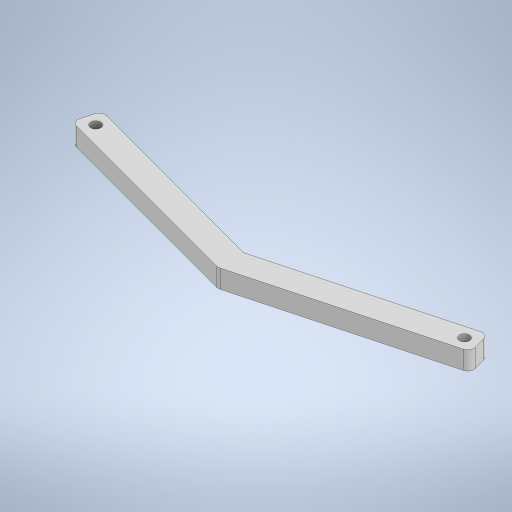
# Autodesk Inventor part: Part3
Saved by Autodesk Inventor 2023 (Build 270158000, 158)
## iProperties
Created: 2023-03-01
Part Number: Part3
Material: Generic
Document SubType Name: Modeling
Designer: Gabriel - T3 CAD
Density: 1 g/cm^3
Appearance: Default
Author: Gabriel - T3 CAD
Autodesk Inventor part; units mm, degrees
ref_plane "YZ Plane" through (0, 0, 0) normal (1, 0, 0) x (0, 1, 0)
ref_plane "XZ Plane" through (0, 0, 0) normal (0, 1, 0) x (-1, 0, 0)
ref_plane "XY Plane" through (0, 0, 0) normal (0, 0, 1) x (1, 0, 0)
sketch "Sketch1" plane through (0, 0, 0) normal (0, 1, 0) x (-1, 0, 0)
  line L0 (0, 0) -> (190.5, 0)
  line L1 (190.5, 0) -> (95.25, 25.5222)
  line L2 (95.25, 25.5222) -> (0, 0)
  line L3 (95.25, 0) -> (95.25, 153.3461)
  line L4 (1.6435, -6.1336) -> (-1.6435, 6.1336)
  line L5 (-1.6435, 6.1336) -> (94.4282, 31.876)
  line L6 (94.4282, 18.728) -> (1.6435, -6.1336)
  line L7 (45.4353, 45.444) -> (42.1483, 33.1767)
  line L8 (96.0718, 18.728) -> (188.8565, -6.1336)
  line L9 (188.8565, -6.1336) -> (192.1435, 6.1336)
  line L10 (192.1435, 6.1336) -> (96.0718, 31.876)
  arc A0 (96.0718, 31.876) -> (94.4282, 31.876) centre (95.25, 28.8092) ccw
  arc A1 (96.0718, 18.728) -> (94.4282, 18.728) centre (95.25, 15.6612) ccw
  circle A2 centre (95.25, 25.5222) radius 2.5797
  circle A3 centre (190.5, 0) radius 2.5797
  circle A4 centre (0, 0) radius 2.5797
  line L11 (192.1435, 6.1336) -> (188.8565, -6.1336)
  line L12 (188.8565, -6.1336) -> (191.9233, -6.9554)
  line L13 (195.8119, -4.7103) -> (197.4554, 1.4233)
  line L14 (195.2103, 5.3119) -> (192.1435, 6.1336)
  arc A5 (197.4554, 1.4233) -> (195.2103, 5.3119) centre (194.3886, 2.2451) ccw
  arc A6 (191.9233, -6.9554) -> (195.8119, -4.7103) centre (192.7451, -3.8886) ccw
  line L15 (-1.6435, 6.1336) -> (1.6435, -6.1336)
  line L16 (1.6435, -6.1336) -> (-1.4233, -6.9554)
  line L17 (-5.3119, -4.7103) -> (-6.9554, 1.4233)
  line L18 (-4.7103, 5.3119) -> (-1.6435, 6.1336)
  arc A7 (-4.7103, 5.3119) -> (-6.9554, 1.4233) centre (-3.8886, 2.2451) ccw
  arc A8 (-5.3119, -4.7103) -> (-1.4233, -6.9554) centre (-2.2451, -3.8886) ccw
  point P0 (95.25, 0)
  point P1 (194.9901, -7.7771)
  point P2 (-4.4901, -7.7771)
  dimension "d0" = 190.5
  dimension "d1" = 150
  dimension "d2" = 12.7
  dimension "d3" = 3.175
  dimension "d4" = 5.1594
  dimension "d6" = 6.35
  dimension "d7" = 3.175
  dimension "d8" = 6.35
  dimension "d9" = 3.175
  constraints: 38 end point, 12 point on circle, 12 tangent, 9 centre point, 9 parallel, 7 point on line, 6 perpendicular, 5 equal radius, 4 coincident, 3 midpoint, 1 collinear, 1 equal length, 1 horizontal
  measures "d0" distance of L0.end L0.start
  measures "d1" angle of L2 L1
  measures "d2" distance of L4.start L4.end
  measures "d3" radius of A0
  measures "d4" diameter of A2
  measures "d6" distance of L8.end point (194.99, -7.777)
  measures "d7" radius of A5
  measures "d8" distance of L4.start point (-4.49, -7.777)
  measures "d9" radius of A7
extrude "Extrusion1" add sketch "Sketch1" along normal blind 9.525 contours A4 L2 A2 L3 A1 L6 L0 | L0 L6 L4 A4 | A4 L4 L5 A0 L3 A2 L2 | L4 L16 A8 L17 A7 L18 A4 | A2 L3 L2 | L2 L3 A2 | L3 A2 L1 | L1 A2 L3 | L3 A0 L10 L9 A3 L1 A2 | A2 L1 A3 L0 L8 A1 L3 | L0 A3 L9 L8 | L9 A3 L14 A5 L13 A6 L12
body "Solid1"
